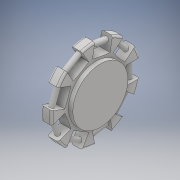
# Autodesk Inventor part: Dasar
Saved by Autodesk Inventor 2017.3 (Build 213257000, 257)
## iProperties
Created: 2020-07-20
Part Number: Dasar
Material: Generic
Document SubType Name: Modeling
Designer: Fahar Endra
Density: 1 g/cm^3
Appearance: Default
Author: Fahar Endra
Autodesk Inventor part; units mm, degrees
ref_plane "YZ Plane" through (0, 0, 0) normal (1, 0, 0) x (0, 1, 0)
ref_plane "XZ Plane" through (0, 0, 0) normal (0, 1, 0) x (-1, 0, 0)
ref_plane "XY Plane" through (0, 0, 0) normal (0, 0, 1) x (1, 0, 0)
sketch "Sketch1" plane through (0, 0, 0) normal (1, 0, 0) x (0, 1, 0)
  circle A0 centre (0, 0) radius 46
  dimension "d8" = 92
  constraints: 1 centre point, 1 coincident
  measures "d8" diameter of A0
extrude "Extrusion1" add sketch "Sketch1" along normal blind 11
sketch "Sketch2" plane through (11, 0, 0) normal (1, 0, 0) x (0, 0, -1)
  point P0 (0, 0)
sketch "Sketch3" plane through (11, 0, 0) normal (1, 0, 0) x (0, 0, -1)
  arc A0 (9.25, 49.1369) -> (-9.25, 49.1369) centre (0, 0) ccw
  line L0 (-9.25, 31) -> (-9.25, 49.1369)
  line L1 (9.25, 31) -> (9.25, 49.1369)
  arc A1 (-9.25, 31) -> (9.25, 31) centre (0, 130.5713) ccw
  constraints: 4 end point, 4 point on circle, 2 centre point, 1 coincident, 1 vertical
extrude "Extrusion2" cut sketch "Sketch3" against normal blind 16
pattern_circular "Circular Pattern1" count 9 over 360 about axis through (0, 0, 0) along (1, 0, 0) of "Extrusion2"
fillet "Fillet1" radius 2 2 edges at (11, 43.2259, 15.7329) (0, 43.2259, 15.7329)
pattern_circular "Circular Pattern2" count 9 over 360 about axis through (0, 0, 0) along (1, 0, 0) of "Fillet1"
sketch "Sketch4" plane through (0, 31, -9.25) normal (0, 0, 1) x (1, 0, 0)
  line L0 (2, 14.0604) -> (2, 9.464) projected
  line L1 (2, 14.0604) -> (9, 14.0604) projected
  line L2 (9, 9.464) -> (9, 14.0604) projected
  line L3 (9, 9.464) -> (2, 9.464) projected
  line L4 (5.5, 14.0604) -> (5.5, 8.5604)
  circle A0 centre (5.5, 8.5604) radius 2.5
  point P0 (0, -31)
  dimension "d23" = 5.5
  dimension "d24" = 5
  constraints: 2 end point, 1 centre point, 1 coincident, 1 midpoint, 1 vertical
  measures "d23" distance of L4.start L4.end
  measures "d24" diameter of A0
extrude "Extrusion3" add sketch "Sketch4" along normal blind 18.5 contours A0 L4 L3 | L3 A0 | A0 L3 L4
pattern_circular "Circular Pattern3" count 9 over 360 about axis through (0, 0, 0) along (1, 0, 0) of "Extrusion3"
sketch "Sketch5" plane through (0, 0, 0) normal (-1, 0, 0) x (0, 0, 1)
  circle A0 centre (0, 0) radius 28.4
  circle A1 centre (0, 0) radius 30.6105
  dimension "d32" = 56.8
  constraints: 2 centre point
  measures "d32" diameter of A0
extrude "Extrusion4" add sketch "Sketch5" along normal blind 3
sketch "Sketch6" plane through (11, 0, 0) normal (1, 0, 0) x (0, 0, -1)
  circle A0 centre (0, 0) radius 28.4
  constraints: 1 centre point, 1 coincident
extrude "Extrusion5" add sketch "Sketch6" along normal blind 4.5
sketch "Sketch7" plane through (0, 0, 0) normal (-1, 0, 0) x (0, 0, 1)
  point P0 (0, 0)
sketch "Sketch8" plane through (0, 0, 0) normal (-1, 0, 0) x (0, 0, 1)
  circle A0 centre (0, 0) radius 14
  dimension "d37" = 28
  constraints: 1 centre point, 1 coincident
  measures "d37" diameter of A0
extrude "Extrusion6" add sketch "Sketch8" along normal blind 3
sketch "Sketch9" plane through (-3, 0, 0) normal (-1, 0, 0) x (0, 0, 1)
  circle A0 centre (0, 0) radius 10.5
  dimension "d40" = 21
  constraints: 1 centre point, 1 coincident
  measures "d40" diameter of A0
extrude "Extrusion7" add sketch "Sketch9" along normal blind 2
body "Solid1"
